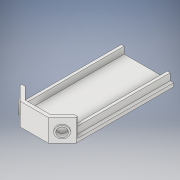
# Autodesk Inventor part: bottom-housing
Saved by Autodesk Inventor 2018 (Build 220112000, 112)
## iProperties
Created: 2019-10-14
Part Number: bottom-housing
Material: Generic
Document SubType Name: Modeling
Designer: jklei
Density: 1 g/cm^3
Appearance: Default
Author: jklei
Autodesk Inventor part; units mm, degrees
ref_plane "YZ Plane" through (0, 0, 0) normal (1, 0, 0) x (0, 1, 0)
ref_plane "XZ Plane" through (0, 0, 0) normal (0, 1, 0) x (-1, 0, 0)
ref_plane "XY Plane" through (0, 0, 0) normal (0, 0, 1) x (1, 0, 0)
sketch "Sketch1" plane through (0, 0, 0) normal (0, 1, 0) x (-1, 0, 0)
  line L0 (0, 0) -> (50.8, 0)
  line L1 (50.8, 0) -> (50.8, -101.6)
  line L2 (50.8, -101.6) -> (0, -101.6)
  line L3 (0, -101.6) -> (0, 0)
  dimension "d0" = 50.8
  dimension "d1" = 101.6
  constraints: 8 end point, 2 parallel, 1 horizontal, 1 perpendicular
  measures "d0" distance of L1.end L2.end
  measures "d1" distance of L0.end L1.end
extrude "Extrusion1" add sketch "Sketch1" along normal blind 3.175
chamfer "Chamfer1" distance 12.7 angle 45 2 edges at (-50.8, 1.5875, 0) (0, 1.5875, 0)
sketch "Sketch3" plane through (0, 3.175, 0) normal (0, 1, 0) x (1, 0, 0)
  line L0 (0, 12.7) -> (-12.7, 0) projected
  line L1 (0, 12.7) -> (0, 101.6) projected
  line L2 (0, 101.6) -> (-50.8, 101.6) projected
  line L3 (-50.8, 101.6) -> (-50.8, 12.7) projected
  line L4 (-38.1, 0) -> (-50.8, 12.7) projected
  line L5 (-38.1, 0) -> (-12.7, 0) projected
  line L6 (-3.175, 14.0151) -> (-14.0151, 3.175)
  line L7 (-14.0151, 3.175) -> (-36.7849, 3.175)
  line L8 (-36.7849, 3.175) -> (-47.625, 14.0151)
  line L9 (-47.625, 14.0151) -> (-50.8, 14.0151)
  line L10 (-3.175, 14.0151) -> (0, 14.0151)
  point P0 (0, 0)
  constraints: 10 end point, 3 point on line, 1 horizontal, 2 other
extrude "Extrusion2" add sketch "Sketch3" along normal blind 17.145 contours L0 L5 L4 L3 L9 L8 L7 L6 L10 L1
sketch "Sketch4" plane through (-12.7, 0, 0) normal (0.7071068, 0, 0.7071068) x (0.7071068, 0, -0.7071068)
  line L0 (0, 20.32) -> (0, 0) projected
  line L1 (0, 0) -> (17.9605, 0) projected
  line L2 (17.9605, 0) -> (17.9605, 20.32) projected
  line L3 (0, 20.32) -> (17.9605, 20.32) projected
  line L4 (16.6454, 20.32) -> (1.3151, 20.32) projected
  line L5 (17.9605, 0) -> (17.9605, 20.32) projected
  line L6 (80.8223, 0) -> (17.9605, 0) projected
  line L7 (80.8223, 0) -> (80.8223, 3.175) projected
  line L8 (18.8904, 3.175) -> (80.8223, 3.175) projected
  line L9 (18.8904, 3.175) -> (18.8904, 20.32) projected
  line L10 (17.9605, 20.32) -> (18.8904, 20.32) projected
  line L11 (16.6454, 3.175) -> (18.8904, 3.175) projected
  line L12 (18.8904, 3.175) -> (17.7679, 3.175)
  line L13 (17.7679, 3.175) -> (0, 3.175)
  line L14 (-14.7855, 3.175) -> (1.3151, 3.175) projected
  circle A0 centre (8.9803, 9.525) radius 4.15
  line L15 (8.9803, 20.32) -> (8.9803, 13.675)
  line L16 (8.9803, 5.375) -> (8.9803, 3.175)
  point P0 (8.9803, 0)
  dimension "d12" = 8.3
  constraints: 8 end point, 3 point on line, 2 midpoint, 2 point on circle, 2 vertical, 1 centre point
  measures "d12" diameter of A0
extrude "Extrusion3" cut sketch "Sketch4" against normal up to next contours A0
sketch "Sketch5" plane through (-50.8, 0, -12.7) normal (-0.7071068, 0, 0.7071068) x (0.7071068, 0, 0.7071068)
  line L0 (0, 20.32) -> (0, 0) projected
  line L1 (-0.9299, 20.32) -> (0, 20.32) projected
  line L2 (-0.9299, 3.175) -> (-0.9299, 20.32) projected
  line L3 (-62.8618, 3.175) -> (-0.9299, 3.175) projected
  line L4 (-62.8618, 0) -> (-62.8618, 3.175) projected
  line L5 (0, 0) -> (-62.8618, 0) projected
  line L6 (0, 20.32) -> (0, 0) projected
  line L7 (0, 0) -> (17.9605, 0) projected
  line L8 (17.9605, 0) -> (17.9605, 20.32) projected
  line L9 (0, 20.32) -> (17.9605, 20.32) projected
  line L10 (-0.9299, 3.175) -> (17.9605, 3.175)
  line L11 (34.9911, 3.175) -> (-26.9408, 3.175) projected
  line L12 (16.6454, 20.32) -> (1.3151, 20.32) projected
  circle A0 centre (8.9803, 9.525) radius 4.15
  line L13 (8.9803, 20.32) -> (8.9803, 13.675)
  line L14 (8.9803, 5.375) -> (8.9803, 3.175)
  point P0 (44.9013, 0)
  dimension "d15" = 8.3
  constraints: 6 end point, 3 point on line, 2 perpendicular, 2 point on circle, 1 centre point, 1 midpoint
  measures "d15" diameter of A0
extrude "Extrusion4" cut sketch "Sketch5" against normal up to next contours A0
sketch "Sketch6" plane through (0, 3.175, 0) normal (0, 1, 0) x (1, 0, 0)
  line L0 (-12.7, 0) -> (0, 12.7) projected
  line L1 (0, 12.7) -> (0, 14.0151) projected
  line L2 (0, 14.0151) -> (-3.175, 14.0151) projected
  line L3 (-3.175, 14.0151) -> (-14.0151, 3.175) projected
  line L4 (-14.0151, 3.175) -> (-36.7849, 3.175) projected
  line L5 (-36.7849, 3.175) -> (-47.625, 14.0151) projected
  line L6 (-47.625, 14.0151) -> (-50.8, 14.0151) projected
  line L7 (-50.8, 14.0151) -> (-50.8, 12.7) projected
  line L8 (-50.8, 12.7) -> (-38.1, 0) projected
  line L9 (-38.1, 0) -> (-12.7, 0) projected
  line L10 (-50.8, 14.0151) -> (-47.625, 14.0151) projected
  line L11 (-47.625, 14.0151) -> (-36.7849, 3.175) projected
  line L12 (-36.7849, 3.175) -> (-14.0151, 3.175) projected
  line L13 (-14.0151, 3.175) -> (-3.175, 14.0151) projected
  line L14 (-3.175, 14.0151) -> (0, 14.0151) projected
  line L15 (0, 14.0151) -> (0, 101.6) projected
  line L16 (0, 101.6) -> (-50.8, 101.6) projected
  line L17 (-50.8, 101.6) -> (-50.8, 14.0151) projected
  line L18 (-3.175, 14.0151) -> (-3.175, 101.6)
  line L19 (-47.625, 14.0151) -> (-47.625, 101.6)
  line L20 (-47.625, 101.6) -> (-45.085, 101.6)
  line L21 (-50.8, 101.6) -> (0, 101.6) projected
  line L22 (-45.085, 101.6) -> (-45.085, 11.4751)
  line L23 (-3.175, 101.6) -> (-5.715, 101.6)
  line L24 (-11.5296, 5.6606) -> (-5.6606, 11.5296) projected
  line L25 (-5.715, 101.6) -> (-5.715, 11.4751)
  point P0 (0, 0)
  dimension "d18" = 2.54
  dimension "d19" = 2.54
  constraints: 12 end point, 6 point on line, 3 vertical, 1 perpendicular
  measures "d18" distance of L19.end L20.end
  measures "d19" distance of L18.end L23.end
extrude "Extrusion5" add sketch "Sketch6" along normal blind 6.35 contours L3 L25 L16 L18 | L19 L16 L22 L5
sketch "Sketch7" plane through (-12.7, 0, 0) normal (0.7071068, 0, 0.7071068) x (0.7071068, 0, -0.7071068)
  circle A0 centre (8.9803, 9.525) radius 4.15 projected
  circle A1 centre (8.9803, 9.525) radius 5.42
  point P0 (8.9803, 0)
  dimension "d22" = 1.27
  constraints: 1 centre point
  measures "d22" radial gap between concentric circles of A0 A1
extrude "Extrusion6" add sketch "Sketch7" along normal blind 1.27
sketch "Sketch8" plane through (-50.8, 0, -12.7) normal (-0.7071068, 0, 0.7071068) x (0.7071068, 0, 0.7071068)
  circle A0 centre (8.9803, 9.525) radius 4.15 projected
  circle A1 centre (8.9803, 9.525) radius 5.42
  point P0 (44.9013, 0)
  dimension "d25" = 1.27
  constraints: 1 centre point
  measures "d25" radial gap between concentric circles of A0 A1
extrude "Extrusion7" add sketch "Sketch8" along normal blind 1.27
body "Solid1"
